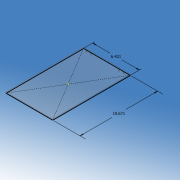
# Autodesk Inventor part: NASA-20-EBOX-LID-REV1-01
Saved by Autodesk Inventor 2020 (Build 240168000, 168)
## iProperties
Created: 2019-09-23
Part Number: NASA-20-EBOX-LID-REV1-01
Material: Polycarbonate, Smoke
Document SubType Name: Modeling
Designer: mpark
Density: 1.2 g/cm^3
Appearance: Polycarbonate - Clear
Mass: 184.217 g
Surface Area: 996.201 cm^2
Volume: 153.514 cm^3
Author: mpark
Title: Electronics Box Lid
Autodesk Inventor part; units mm, degrees
ref_plane "YZ Plane" through (0, 0, 0) normal (1, 0, 0) x (0, 1, 0)
ref_plane "XZ Plane" through (0, 0, 0) normal (0, 1, 0) x (-1, 0, 0)
ref_plane "XY Plane" through (0, 0, 0) normal (0, 0, 1) x (1, 0, 0)
sketch "Sketch1" plane through (0, 0, 0) normal (0, 1, 0) x (-1, 0, 0)
  line L0 (107.95, 174.625) -> (-107.95, 174.625)
  line L1 (-107.95, 174.625) -> (-107.95, -174.625)
  line L2 (-107.95, -174.625) -> (107.95, -174.625)
  line L3 (107.95, -174.625) -> (107.95, 174.625)
  line L4 (107.95, 174.625) -> (-107.95, -174.625) construction
  line L5 (-107.95, 174.625) -> (107.95, -174.625) construction
  point P0 (0, 0)
  dimension "d0" = 215.9
  dimension "d1" = 349.25
  constraints: 12 end point, 2 midpoint, 2 parallel, 1 horizontal, 1 perpendicular
  measures "d0" distance of L2.end L1.end
  measures "d1" distance of L1.end L0.end
extrude "Extrusion1" add sketch "Sketch1" along normal blind 3.175
body "Solid1"
